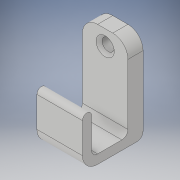
# Autodesk Inventor part: hook_straight
Saved by Autodesk Inventor 2019 (Build 230136000, 136)
## iProperties
Created: 2019-02-20
Part Number: hook_straight
Material: Generic
Document SubType Name: Modeling
Designer: jmc
Density: 1 g/cm^3
Appearance: Default
Author: jmc
Autodesk Inventor part; units mm, degrees
ref_plane "YZ Plane" through (0, 0, 0) normal (1, 0, 0) x (0, 1, 0)
ref_plane "XZ Plane" through (0, 0, 0) normal (0, 1, 0) x (-1, 0, 0)
ref_plane "XY Plane" through (0, 0, 0) normal (0, 0, 1) x (1, 0, 0)
sketch "Sketch1" plane through (0, 0, 0) normal (0, 0, 1) x (1, 0, 0)
  line L0 (-2.5, 15) -> (2.5, 15)
  line L1 (7.5, 10) -> (7.5, -15)
  line L2 (7.5, -15) -> (-7.5, -15)
  line L3 (-7.5, -15) -> (-7.5, 10)
  line L4 (-7.5, 15) -> (7.5, -15) construction
  line L5 (7.5, 15) -> (-7.5, -15) construction
  arc A0 (-2.5, 15) -> (-7.5, 10) centre (-2.5, 10) ccw
  arc A1 (7.5, 10) -> (2.5, 15) centre (2.5, 10) ccw
  circle A2 centre (0, 10) radius 1.5
  point P0 (0, 0)
  dimension "d0" = 15
  dimension "HOOK_LEN" = 30
  dimension "d2" = 5
  dimension "d3" = 3
  dimension "d13" = 5
  constraints: 12 end point, 4 point on circle, 4 point on line, 4 tangent, 3 centre point, 2 midpoint, 2 parallel, 1 equal radius, 1 horizontal, 1 perpendicular
  measures "d0" distance of L1.end L2.end
  measures "HOOK_LEN" distance of L5.start L1.end
  measures "d2" radius of A0
  measures "d3" diameter of A2
  measures "d13" distance from line of L0 A2.centre
extrude "Extrusion1" add sketch "Sketch1" along normal blind 5
sketch "Sketch2" plane through (0, 0, 5) normal (0, 0, 1) x (1, 0, 0)
  circle A0 centre (0, 10) radius 1.5 projected
  point P0 (0, 0)
  point P1 (0, 10)
  constraints: 1 coincident
hole "Hole1" at (0, 10, 5) direction (0, 0, -1) diameter 4 end through all countersink diameter 6 countersink angle 90
sketch "Sketch3" plane through (-7.5, -15, 0) normal (-1, 0, 0) x (0, 0, 1)
  line L0 (5, 0) -> (15, 0)
  arc A0 (15, 0) -> (20, 5) centre (15, 5) ccw
  line L1 (20, 5) -> (20, 15)
  line L2 (20, 15) -> (20, 5)
  arc A1 (15, 3) -> (17, 5) centre (15, 5) ccw
  line L3 (15, 3) -> (7, 3)
  line L4 (17, 5) -> (17, 15)
  arc A2 (20, 15) -> (17, 15) centre (18.5, 15) ccw
  arc A3 (5, 5) -> (7, 3) centre (7, 5) ccw
  line L5 (5, 25) -> (5, 0) projected
  line L6 (5, 5) -> (5, 0)
  point P0 (0, 15)
  dimension "d14" = 10
  dimension "d15" = 10
  dimension "d17" = 3
  dimension "d19" = 4
  constraints: 12 end point, 8 point on circle, 5 tangent, 4 centre point, 2 collinear, 2 vertical, 1 horizontal
  measures "d14" distance of L0.start L0.end
  measures "d15" diameter of A0
  measures "d17" radial gap between concentric circles of A0 A1
  measures "d19" diameter of A3
extrude "Extrusion2" add sketch "Sketch3" against normal up to surface (15 mm away)
sketch "Sketch4" plane through (-7.5, -15, 0) normal (-1, 0, 0) x (0, 0, 1)
  arc A0 (0, 2) -> (2, 0) centre (2, 2) ccw
  line L0 (0, 25) -> (0, 0) projected
  line L1 (0, 0) -> (15, 0) projected
  point P0 (0, 15)
  dimension "d22" = 4
  constraints: 2 point on circle, 2 point on line, 2 tangent, 1 centre point
  measures "d22" diameter of A0
extrude "Extrusion3" cut sketch "Sketch4" against normal through all
body "Solid1"
